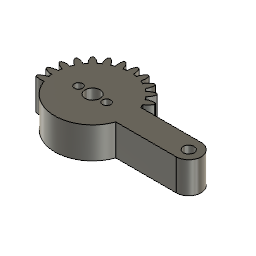
Gear (Autodesk Fusion 360 design; units mm, degrees)
part number: 2026-08-19-19-26-28-269
Autodesk Fusion 360 part; units mm, degrees
note: some values were not read from the file. Set by a fixed rule: which sketch regions a step uses.
sketch "Sketch1" plane through (0, 0, 0) normal (0, 0, 1) x (1, 0, 0)
  circle A0 centre (0, 0) radius 12.09
  line L0 (0, 0) -> (30.75, 0)
  circle A1 centre (30.75, 0) radius 1.75
  circle A2 centre (0, 0) radius 1.75
  line L1 (0, -14.63) -> (0, 14.63) construction
  line L2 (0, 14.63) -> (-0.31, 14.63)
  line L3 (0, 14.63) -> (-0.31, 14.63)
  arc A3 (-0.31, 14.63) -> (-1.04, 12.0452) centre (3.9012, 12.0452) ccw
  arc A4 (1.04, 12.0452) -> (0.31, 14.63) centre (-3.9012, 12.0452) ccw
  line L4 (0.31, 14.63) -> (0, 14.63)
  arc A5 (-4.086, 14.0513) -> (-4.1221, 11.3656) centre (0.6508, 12.6445) ccw
  line L5 (-3.7865, 14.1315) -> (-4.086, 14.0513)
  line L6 (-3.4871, 14.2117) -> (-3.7865, 14.1315)
  arc A6 (-2.113, 11.9039) -> (-3.4871, 14.2117) centre (-6.8858, 10.625) ccw
  arc A7 (-7.5835, 12.515) -> (-6.9233, 9.9114) centre (-2.644, 12.382) ccw
  line L7 (-7.315, 12.67) -> (-7.5835, 12.515)
  line L8 (-7.0465, 12.825) -> (-7.315, 12.67)
  arc A8 (-5.1219, 10.9514) -> (-7.0465, 12.825) centre (-9.4011, 8.4808) ccw
  arc A9 (-10.5642, 10.1258) -> (-9.2526, 7.7818) centre (-5.7587, 11.2758) ccw
  line L9 (-10.345, 10.345) -> (-10.5642, 10.1258)
  line L10 (-10.1258, 10.5642) -> (-10.345, 10.345)
  arc A10 (-7.7818, 9.2526) -> (-10.1258, 10.5642) centre (-11.2758, 5.7587) ccw
  arc A11 (-12.825, 7.0465) -> (-10.9514, 5.1219) centre (-8.4808, 9.4011) ccw
  line L11 (-12.67, 7.315) -> (-12.825, 7.0465)
  line L12 (-12.515, 7.5835) -> (-12.67, 7.315)
  arc A12 (-9.9114, 6.9233) -> (-12.515, 7.5835) centre (-12.382, 2.644) ccw
  arc A13 (-14.2117, 3.4871) -> (-11.9039, 2.113) centre (-10.625, 6.8858) ccw
  line L13 (-14.1315, 3.7865) -> (-14.2117, 3.4871)
  line L14 (-14.0513, 4.086) -> (-14.1315, 3.7865)
  arc A14 (-11.3656, 4.1221) -> (-14.0513, 4.086) centre (-12.6445, -0.6508) ccw
  arc A15 (-14.63, -0.31) -> (-12.0452, -1.04) centre (-12.0452, 3.9012) ccw
  line L15 (-14.63, 0) -> (-14.63, -0.31)
  line L16 (-14.63, 0.31) -> (-14.63, 0)
  arc A16 (-12.0452, 1.04) -> (-14.63, 0.31) centre (-12.0452, -3.9012) ccw
  arc A17 (-14.0513, -4.086) -> (-11.3656, -4.1221) centre (-12.6445, 0.6508) ccw
  line L17 (-14.1315, -3.7865) -> (-14.0513, -4.086)
  line L18 (-14.2117, -3.4871) -> (-14.1315, -3.7865)
  arc A18 (-11.9039, -2.113) -> (-14.2117, -3.4871) centre (-10.625, -6.8858) ccw
  arc A19 (12.515, 7.5835) -> (9.9114, 6.9233) centre (12.382, 2.644) ccw
  line L19 (12.67, 7.315) -> (12.515, 7.5835)
  line L20 (12.825, 7.0465) -> (12.67, 7.315)
  arc A20 (10.9514, 5.1219) -> (12.825, 7.0465) centre (8.4808, 9.4011) ccw
  arc A21 (10.1258, 10.5642) -> (7.7818, 9.2526) centre (11.2758, 5.7587) ccw
  line L21 (10.345, 10.345) -> (10.1258, 10.5642)
  line L22 (10.5642, 10.1258) -> (10.345, 10.345)
  arc A22 (9.2526, 7.7818) -> (10.5642, 10.1258) centre (5.7587, 11.2758) ccw
  arc A23 (7.0465, 12.825) -> (5.1219, 10.9514) centre (9.4011, 8.4808) ccw
  line L23 (7.315, 12.67) -> (7.0465, 12.825)
  line L24 (7.5835, 12.515) -> (7.315, 12.67)
  arc A24 (6.9233, 9.9114) -> (7.5835, 12.515) centre (2.644, 12.382) ccw
  arc A25 (3.4871, 14.2117) -> (2.113, 11.9039) centre (6.8858, 10.625) ccw
  line L25 (3.7865, 14.1315) -> (3.4871, 14.2117)
  line L26 (4.086, 14.0513) -> (3.7865, 14.1315)
  arc A26 (4.1221, 11.3656) -> (4.086, 14.0513) centre (-0.6508, 12.6445) ccw
  circle A27 centre (30.75, 0) radius 4
  line L27 (30.75, 4) -> (11.4091, 4)
  line L28 (30.75, -4) -> (11.4091, -4)
  dimension "d1" = 24.18
  dimension "d2" = 30.75
  dimension "d3" = 3.5
  dimension "d4" = 3.5
  dimension "d5" = 29.26
  dimension "d6" = 0.31
  dimension "d9" = 360
  dimension "d10" = 8
  constraint coincident A0.centre L0.start
  constraint horizontal L0
  constraint coincident L0.end A1.centre
  constraint midpoint L1 A0.centre
  constraint perpendicular L0 L1
  constraint perpendicular L1 L2
  constraint perpendicular L1 L3
  constraint coincident A0 A3.end
  constraint symmetric L1 L2.end A4.end
  constraint symmetric L1 A3.end A4.start
  constraint symmetric L1 A3 A4
  constraint concentric A1 A27
  constraint coincident A27 L27.start
  constraint coincident A0 L27.end
  constraint tangent A27 L27
  constraint horizontal L27
  constraint coincident A27 L28.start
  constraint coincident A0 L28.end
  constraint tangent A27 L28
  constraint parallel L27 L28
  measures "d1" diameter of A0
  measures "d2" distance of A0.centre L0.end
  measures "d3" diameter of A1
  measures "d4" diameter of A2
  measures "d5" distance of L1.start L1.end
  measures "d6" distance of L1.end L2.end
  measures "d10" diameter of A27
extrude "Extrude1" add sketch "Sketch1" along normal blind 10
sketch "Sketch2" plane through (0, 0, 10) normal (0, 0, 1) x (-1, 0, 0)
  circle A0 centre (-30.75, 0) radius 1.75
  circle A1 centre (0, 0) radius 1.75
  line L0 (-30.75, -4) -> (-11.4091, -4)
  arc A2 (-11.4091, -4) -> (-10.9514, -5.1219) centre (0, 0) ccw
  arc A3 (-10.9514, -5.1219) -> (-12.825, -7.0465) centre (-8.4808, -9.4011) ccw
  line L1 (-12.825, -7.0465) -> (-12.515, -7.5835)
  arc A4 (-12.515, -7.5835) -> (-9.9114, -6.9233) centre (-12.382, -2.644) ccw
  arc A5 (-9.9114, -6.9233) -> (-9.2526, -7.7818) centre (0, 0) ccw
  arc A6 (-9.2526, -7.7818) -> (-10.5642, -10.1258) centre (-5.7587, -11.2758) ccw
  line L2 (-10.5642, -10.1258) -> (-10.1258, -10.5642)
  arc A7 (-10.1258, -10.5642) -> (-7.7818, -9.2526) centre (-11.2758, -5.7587) ccw
  arc A8 (-7.7818, -9.2526) -> (-6.9233, -9.9114) centre (0, 0) ccw
  arc A9 (-6.9233, -9.9114) -> (-7.5835, -12.515) centre (-2.644, -12.382) ccw
  line L3 (-7.5835, -12.515) -> (-7.0465, -12.825)
  arc A10 (-7.0465, -12.825) -> (-5.1219, -10.9514) centre (-9.4011, -8.4808) ccw
  arc A11 (-5.1219, -10.9514) -> (-4.1221, -11.3656) centre (0, 0) ccw
  arc A12 (-4.1221, -11.3656) -> (-4.086, -14.0513) centre (0.6508, -12.6445) ccw
  line L4 (-4.086, -14.0513) -> (-3.4871, -14.2117)
  arc A13 (-3.4871, -14.2117) -> (-2.113, -11.9039) centre (-6.8858, -10.625) ccw
  arc A14 (-2.113, -11.9039) -> (-1.04, -12.0452) centre (0, 0) ccw
  arc A15 (-1.04, -12.0452) -> (-0.31, -14.63) centre (3.9012, -12.0452) ccw
  line L5 (-0.31, -14.63) -> (0.31, -14.63)
  arc A16 (0.31, -14.63) -> (1.04, -12.0452) centre (-3.9012, -12.0452) ccw
  arc A17 (1.04, -12.0452) -> (2.113, -11.9039) centre (0, 0) ccw
  arc A18 (2.113, -11.9039) -> (3.4871, -14.2117) centre (6.8858, -10.625) ccw
  line L6 (3.4871, -14.2117) -> (4.086, -14.0513)
  arc A19 (4.086, -14.0513) -> (4.1221, -11.3656) centre (-0.6508, -12.6445) ccw
  arc A20 (4.1221, -11.3656) -> (5.1219, -10.9514) centre (0, 0) ccw
  arc A21 (5.1219, -10.9514) -> (7.0465, -12.825) centre (9.4011, -8.4808) ccw
  line L7 (7.0465, -12.825) -> (7.5835, -12.515)
  arc A22 (7.5835, -12.515) -> (6.9233, -9.9114) centre (2.644, -12.382) ccw
  arc A23 (6.9233, -9.9114) -> (7.7818, -9.2526) centre (0, 0) ccw
  arc A24 (7.7818, -9.2526) -> (10.1258, -10.5642) centre (11.2758, -5.7587) ccw
  line L8 (10.1258, -10.5642) -> (10.5642, -10.1258)
  arc A25 (10.5642, -10.1258) -> (9.2526, -7.7818) centre (5.7587, -11.2758) ccw
  arc A26 (9.2526, -7.7818) -> (9.9114, -6.9233) centre (0, 0) ccw
  arc A27 (9.9114, -6.9233) -> (12.515, -7.5835) centre (12.382, -2.644) ccw
  line L9 (12.515, -7.5835) -> (12.825, -7.0465)
  arc A28 (12.825, -7.0465) -> (10.9514, -5.1219) centre (8.4808, -9.4011) ccw
  arc A29 (10.9514, -5.1219) -> (11.3656, -4.1221) centre (0, 0) ccw
  arc A30 (11.3656, -4.1221) -> (14.0513, -4.086) centre (12.6445, 0.6508) ccw
  line L10 (14.0513, -4.086) -> (14.2117, -3.4871)
  arc A31 (14.2117, -3.4871) -> (11.9039, -2.113) centre (10.625, -6.8858) ccw
  arc A32 (11.9039, -2.113) -> (12.0452, -1.04) centre (0, 0) ccw
  arc A33 (12.0452, -1.04) -> (14.63, -0.31) centre (12.0452, 3.9012) ccw
  line L11 (14.63, -0.31) -> (14.63, 0.31)
  arc A34 (14.63, 0.31) -> (12.0452, 1.04) centre (12.0452, -3.9012) ccw
  arc A35 (12.0452, 1.04) -> (11.9039, 2.113) centre (0, 0) ccw
  arc A36 (11.9039, 2.113) -> (14.2117, 3.4871) centre (10.625, 6.8858) ccw
  line L12 (14.2117, 3.4871) -> (14.0513, 4.086)
  arc A37 (14.0513, 4.086) -> (11.3656, 4.1221) centre (12.6445, -0.6508) ccw
  arc A38 (11.3656, 4.1221) -> (-11.4091, 4) centre (0, 0) ccw
  line L13 (-11.4091, 4) -> (-30.75, 4)
  arc A39 (-30.75, 4) -> (-30.75, -4) centre (-30.75, 0) ccw
  line L14 (4.5, 0) -> (-4.5, 0) construction
  circle A40 centre (4.5, 0) radius 1.3
  circle A41 centre (-4.5, 0) radius 1.3
  dimension "d13" = 9
  dimension "d14" = 2.6
  dimension "d15" = 2.6
  constraint midpoint L14 A1.centre
  constraint coincident A1.centre A2.centre
  constraint horizontal L14
  constraint coincident L14.start A40.centre
  constraint coincident L14.end A41.centre
  measures "d13" distance of L14.start L14.end
  measures "d14" diameter of A40
  measures "d15" diameter of A41
sketch "Sketch3" plane through (0, 0, 10) normal (0, 0, 1) x (-1, 0, 0)
extrude "Extrude2" cut sketch "Sketch2" against normal blind 10 contours A40
extrude "Extrude3" cut sketch "Sketch2" against normal blind 10 contours A41
sketch "Sketch4" plane through (0, 0, 10) normal (0, 0, 1) x (-1, 0, 0)
  circle A0 centre (0, 0) radius 2.4
  dimension "d20" = 4.8
  constraint coincident A0.centre origin
  measures "d20" diameter of A0
extrude "Extrude4" cut sketch "Sketch4" against normal blind 10
